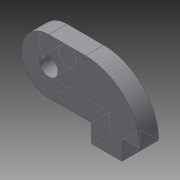
# Autodesk Inventor part: Bottom battery holder
Saved by Autodesk Inventor 2015 (Build 190159000, 159)
## iProperties
Created: 2014-11-12
Part Number: Bottom battery holder
Material: Generic
Document SubType Name: Modeling
Designer: karl
Density: 1 g/cm^3
Appearance: Default
Author: karl
Autodesk Inventor part; units mm, degrees
ref_plane "YZ Plane" through (0, 0, 0) normal (1, 0, 0) x (0, 1, 0)
ref_plane "XZ Plane" through (0, 0, 0) normal (0, 1, 0) x (-1, 0, 0)
ref_plane "XY Plane" through (0, 0, 0) normal (0, 0, 1) x (1, 0, 0)
sketch "Sketch1" plane through (0, 0, 0) normal (0, 1, 0) x (-1, 0, 0)
  line L0 (-7.5, -4.5) -> (7.5, -4.5)
  line L1 (7.5, -4.5) -> (7.5, 4.5)
  line L2 (7.5, 4.5) -> (-7.5, 4.5)
  line L3 (-7.5, 4.5) -> (-7.5, -4.5)
  line L4 (-7.5, -4.5) -> (7.5, 4.5) construction
  line L5 (7.5, -4.5) -> (-7.5, 4.5) construction
  circle A0 centre (7.5, 0) radius 1.5
  circle A1 centre (7.5, 0) radius 4.5
  point P0 (0, 0)
  dimension "d0" = 15
  dimension "d1" = 3
  dimension "d2" = 9
  dimension "d3" = 9
  constraints: 12 end point, 3 midpoint, 2 centre point, 2 parallel, 1 coincident, 1 horizontal, 1 perpendicular, 1 tangent
  measures "d0" distance of L2.end L1.end
  measures "d1" diameter of A0
  measures "d2" distance between parallel lines of L0 L2
  measures "d3" diameter of A1
extrude "Extrusion1" add sketch "Sketch1" along normal blind 3 contours L3 L2 A1 L0 | A1 L1 A0 | L1 A0 A1 | A0 L1 picked at (7.0325, 0.1773)
sketch "Sketch2" plane through (0, 3, 0) normal (0, 1, 0) x (1, 0, 0)
  line L0 (-7.5, -1.5) -> (-7.5, 1.5) projected
  circle A0 centre (-7.5, 0) radius 1.5
  point P0 (0, 0)
  dimension "d6" = 3
  constraints: 1 centre point, 1 midpoint
  measures "d6" diameter of A0
extrude "Extrusion2" cut sketch "Sketch2" against normal blind 3
sketch "Sketch3" plane through (0, 3, 0) normal (0, 1, 0) x (1, 0, 0)
  line L0 (7.5, 4.5) -> (-7.5, 4.5) projected
  line L1 (4.5, 4.5) -> (-0.5, 4.5)
  line L2 (-0.5, 4.5) -> (-0.5, 7.5)
  line L3 (-0.5, 7.5) -> (4.5, 7.5)
  line L4 (4.5, 7.5) -> (4.5, 4.5)
  line L5 (7.5, -4.5) -> (7.5, 4.5) projected
  point P0 (0, 0)
  dimension "d9" = 5
  dimension "d10" = 3
  dimension "d11" = 3
  constraints: 8 end point, 2 parallel, 1 horizontal, 1 perpendicular, 1 point on line
  measures "d9" distance of L2.end L3.end
  measures "d10" distance of L1.end L2.end
  measures "d11" distance between parallel lines of L5 L4
extrude "Extrusion3" add sketch "Sketch3" against normal blind 3
fillet "Fillet1" radius 9 1 edges at (7.5, 1.5, 4.5)
body "Solid1"
